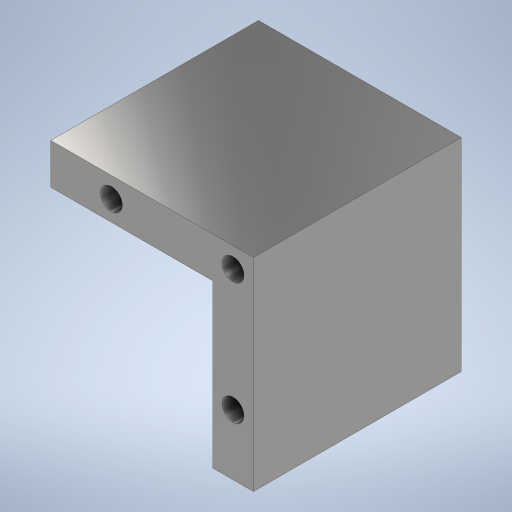
# Autodesk Inventor part: MirroHouseModel
Saved by Autodesk Inventor 2023 (Build 270158000, 158)
## iProperties
Created: 2022-10-18
Part Number: MirroHouseModel
Material: Steel, Carbon
Document SubType Name: Modeling
Designer: Miner
Density: 7.85 g/cm^3
Appearance: Semi-Polished
Author: Miner
Autodesk Inventor part; units mm, degrees
ref_plane "YZ Plane" through (0, 0, 0) normal (1, 0, 0) x (0, 1, 0)
ref_plane "XZ Plane" through (0, 0, 0) normal (0, 1, 0) x (-1, 0, 0)
ref_plane "XY Plane" through (0, 0, 0) normal (0, 0, 1) x (1, 0, 0)
sketch "Sketch1" plane through (0, 0, 0) normal (0, 0, 1) x (1, 0, 0)
  line L0 (20, -20) -> (20, 20) construction
  line L1 (20, 20) -> (-20, 20) construction
  line L2 (-20, 20) -> (-20, -20) construction
  line L3 (-20, -20) -> (20, 20) construction
  line L4 (20, -20) -> (-20, 20) construction
  line L5 (20, 20) -> (-20, 20)
  line L6 (20, 20) -> (20, -20)
  line L7 (-20, -20) -> (20, -20) construction
  line L8 (20, -20) -> (12, -20)
  line L9 (12, -20) -> (12, 12)
  line L10 (12, 12) -> (-20, 12)
  line L11 (-20, 20) -> (-20, 12)
  point P0 (0, 0)
  dimension "d0" = 40
  dimension "d1" = 40
  dimension "d3" = 8
  constraints: 24 end point, 3 perpendicular, 3 point on line, 2 midpoint, 1 collinear, 1 parallel
  measures "d0" distance of L1.end L0.end
  measures "d1" distance of L0.end L0.start
  measures "d3" distance of L7.end L8.end
extrude "Extrusion1" add sketch "Sketch1" along normal blind 41
sketch "Sketch2" plane through (0, 0, 41) normal (0, 0, 1) x (1, 0, 0)
  line L0 (20, 20) -> (-20, 20) construction
  line L1 (20, 20) -> (20, 16) construction
  line L2 (20, -20) -> (20, 20) construction
  line L3 (20, 16) -> (16, 16) construction
  line L4 (16, 16) -> (-8, 16) construction
  line L5 (16, 16) -> (16, -8) construction
  point P0 (0, 0)
  dimension "d6" = 4
  dimension "d7" = 4
  dimension "d8" = 24
  dimension "d9" = 24
  constraints: 8 end point, 3 coincident, 2 perpendicular, 2 point on line
  measures "d6" distance of L0.start L1.end
  measures "d7" distance of L1.end L3.end
  measures "d8" distance of L3.end L4.end
  measures "d9" distance of L3.end L5.end
hole "Hole1" at (-8, 16, 41) at (16, 16, 41) at (16, -8, 41) direction (0, 0, -1) diameter 4.3 depth 5 tip angle 118
body "Solid1"
